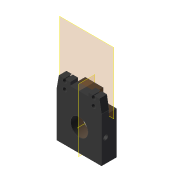
# Autodesk Inventor part: 30_Cube_Z_Focus_MGN_NEMA_adapter_M12
Saved by Autodesk Inventor 2019.4 (Build 234330000, 330)
## iProperties
Created: 2021-04-25
Part Number: 30_Cube_Z_Focus_MGN_NEMA_adapter_M12
Material: Generic
Document SubType Name: Modeling
Designer: diederichbenedict
Density: 1 g/cm^3
Appearance: Default
Author: diederichbenedict
Autodesk Inventor part; units mm, degrees
note: some values were not read from the file. Chosen so that the rebuilt part matches the saved one: sketch regions of "Extrusion1".
ref_plane "YZ Plane" through (0, 0, 0) normal (1, 0, 0) x (0, 1, 0)
ref_plane "XZ Plane" through (0, 0, 0) normal (0, 1, 0) x (-1, 0, 0)
ref_plane "XY Plane" through (0, 0, 0) normal (0, 0, 1) x (1, 0, 0)
ref_plane "Work Plane1" through (0, 0, 0) normal (0, 0, 1) x (1, 0, 0)
sketch "Sketch1" plane through (0, 0, 0) normal (0, 0, 1) x (1, 0, 0)
  circle A0 centre (6.843, -28.9967) radius 1.4 projected
  circle A1 centre (26.1569, -28.9967) radius 1.4 projected
  circle A2 centre (26.1569, -23.9967) radius 1.4 projected
  circle A3 centre (6.843, -23.9967) radius 1.4 projected
  line L0 (0.4643, -12) -> (0, -12) construction
  line L1 (3.1567, -14.6923) -> (0.4643, -12) construction
  line L2 (3.1567, -32.6831) -> (3.1567, -14.6923) construction
  line L3 (10.5294, -32.6831) -> (3.1567, -32.6831) projected
  line L4 (10.5294, -14.6923) -> (10.5294, -32.6831) construction
  line L5 (9, -11) -> (10.5294, -14.6923) construction
  line L6 (2.8, -11) -> (9, -11) construction
  line L7 (2.8, 0) -> (2.8, -11) construction
  line L8 (30.2, 0) -> (2.8, 0) construction
  line L9 (30.2, 0) -> (30.2, -11) construction
  line L10 (24, -11) -> (30.2, -11) construction
  line L11 (24, -11) -> (22.4706, -14.6923) construction
  line L12 (22.4706, -14.6923) -> (22.4706, -32.6831) construction
  line L13 (22.4706, -32.6831) -> (29.8433, -32.6831) projected
  line L14 (29.8433, -32.6831) -> (29.8433, -14.6923) construction
  line L15 (29.8433, -14.6923) -> (32.5357, -12) construction
  line L16 (33, -12) -> (32.5357, -12) construction
  line L17 (33, -12) -> (33, 5) construction
  line L18 (0, 5) -> (0, -12) construction
  circle A4 centre (16.4744, -46.03) radius 10 projected
  circle A5 centre (16.4744, -46.03) radius 12.5
  line L19 (31.4744, -31.03) -> (1.4744, -31.03) construction
  line L20 (1.4744, -31.03) -> (1.4744, -61.03) construction
  line L21 (1.4744, -61.03) -> (31.4744, -61.03) construction
  line L22 (31.4744, -61.03) -> (31.4744, -31.03) construction
  line L23 (31.4744, -31.03) -> (1.4744, -61.03) construction
  line L24 (1.4744, -31.03) -> (31.4744, -61.03) construction
  line L25 (31.4744, -61.03) -> (1.4744, -61.03)
  line L26 (1.4744, -61.03) -> (1.4744, -31.03)
  line L27 (1.4744, -31.03) -> (31.4744, -31.03)
  line L28 (31.4744, -31.03) -> (31.4744, -61.03)
  line L29 (31.4744, -61.03) -> (1.4744, -31.03) construction
  line L30 (1.4744, -61.03) -> (31.4744, -31.03) construction
  line L31 (1.4744, -31.03) -> (3.1567, -21.6555)
  line L32 (3.1567, -21.6555) -> (29.8433, -21.6555)
  line L33 (31.4744, -31.03) -> (29.8433, -21.6555)
  circle A6 centre (15.4444, 14.8) radius 2 projected
  line L34 (19.4444, 18.8) -> (33, 5) projected
  line L35 (11.4444, 18.8) -> (19.4444, 18.8) projected
  line L36 (0, 5) -> (11.4444, 18.8) projected
  circle A7 centre (3.9444, 3.3) radius 1.45 projected
  circle A8 centre (26.9444, 3.3) radius 1.45 projected
  point P0 (0, 0)
  dimension "d0" = 25
  dimension "d1" = 30
  dimension "d2" = 30
  constraints: 30 end point, 4 midpoint, 4 parallel, 3 perpendicular, 2 horizontal, 2 point on line, 1 centre point, 1 coincident
  measures "d0" diameter of A5
  measures "d1" distance of L21.end L20.end
  measures "d2" distance of L20.end L19.end
extrude "Extrusion1" add sketch "Sketch1" along normal blind 5 contours L25 L26 L27 L28 | L27 L31 L32 L33
sketch "Sketch2" plane through (0, 0, 0) normal (0, 0, -1) x (-1, 0, 0)
  circle A0 centre (-16.4744, -46.03) radius 12.5 projected
  circle A1 centre (-16.4744, -46.03) radius 10.5
  line L0 (0.4956, -63) -> (-33.4444, -63) projected
  circle A2 centre (-16.4744, -46.03) radius 12.5 projected
  arc A3 (-23.9744, -56.03) -> (-8.9744, -56.03) centre (-16.4744, -46.03) ccw
  arc A4 (-21.3847, -34.5348) -> (-28.8847, -47.5252) centre (-16.4744, -46.03) ccw
  arc A5 (-4.0642, -47.5252) -> (-11.5642, -34.5348) centre (-16.4744, -46.03) ccw
  point P0 (0, 0)
  dimension "d5" = 21
  constraints: 12 point on circle, 4 centre point, 2 coincident, 3 other
  measures "d5" diameter of A1
extrude "Extrusion2" add sketch "Sketch2" against normal up to surface (5 mm away)
sketch "Sketch3" plane through (0, 0, 0) normal (0, 0, -1) x (-1, 0, 0)
  line L0 (-30.5357, -14) -> (-24, -14) construction
  line L1 (-30.5357, -14) -> (-29.8433, -14.6923) construction
  line L2 (-29.8433, -14.6923) -> (-29.8433, -32.6831) construction
  line L3 (-29.8433, -32.6831) -> (-22.4706, -32.6831) projected
  line L4 (-22.4706, -32.6831) -> (-10.5294, -32.6831)
  line L5 (-10.5294, -32.6831) -> (-10.5294, -22.0651)
  line L6 (-10.5294, -22.0651) -> (-22.4706, -22.0651)
  line L7 (-22.4706, -22.0651) -> (-22.4706, -32.6831)
  circle A0 centre (-6.843, -23.9967) radius 1.4 construction
  circle A1 centre (-26.1569, -23.9967) radius 1.4 construction
  circle A2 centre (-26.1569, -28.9967) radius 1.4 construction
  circle A3 centre (-6.843, -28.9967) radius 1.4 construction
  line L8 (-3.1567, -21.6555) -> (-1.4744, -31.03) construction
  line L9 (-29.8433, -21.6555) -> (-3.1567, -21.6555) construction
  line L10 (-31.4744, -31.03) -> (-29.8433, -21.6555) construction
  line L11 (-31.4744, -61.03) -> (-31.4744, -31.03) construction
  line L12 (-1.4744, -61.03) -> (-31.4744, -61.03) projected
  line L13 (-1.4744, -31.03) -> (-1.4744, -61.03) construction
  line L14 (-31.4744, -32.6831) -> (-29.8433, -32.6831)
  line L15 (-3.1567, -32.6831) -> (-1.4744, -32.6831)
  line L16 (-31.4744, -61.03) -> (-1.4744, -61.03)
  line L17 (-1.4744, -61.03) -> (-1.4744, -32.6831)
  line L18 (-1.4744, -32.6831) -> (-31.4744, -32.6831)
  line L19 (-31.4744, -32.6831) -> (-31.4744, -61.03)
  circle A4 centre (-26.1569, -28.9967) radius 1.4 projected
  circle A5 centre (-26.1569, -23.9967) radius 1.4 projected
  line L20 (-24, -14) -> (-24, -11) projected
  line L21 (-22.4706, -32.6831) -> (-22.4706, -14.6923) projected
  line L22 (-22.4706, -14.6923) -> (-24, -11) projected
  circle A6 centre (-16.4256, -45.91) radius 10.6939 projected
  point P0 (0, 0)
  constraints: 20 end point, 4 parallel, 4 point on line, 2 horizontal, 2 perpendicular, 1 collinear
extrude "Extrusion4" add sketch "Sketch3" along normal blind 5 contours L3 L4 L18 L15 L17 L12 L19 L14 | L7 L6 L5 L4
sketch "Sketch4" plane through (3.1567, -21.6555, 0) normal (0, 1, 0) x (1, 0, 0)
  line L0 (-6.8596, 8.2929) -> (32.2101, 8.2929)
  line L1 (32.2101, 8.2929) -> (32.2101, -9.1799)
  line L2 (32.2101, -9.1799) -> (-6.8596, -9.1799)
  line L3 (-6.8596, -9.1799) -> (-6.8596, 8.2929)
  point P0 (-3.1567, 0)
  constraints: 8 end point, 2 parallel, 1 horizontal, 1 perpendicular
extrude "Extrusion5" cut sketch "Sketch4" against normal blind 1
sketch "Sketch5" plane through (0, 0, 5) normal (0, 0, 1) x (1, 0, 0)
  circle A0 centre (6.843, -28.9967) radius 1.4 projected
  circle A1 centre (26.1569, -28.9967) radius 1.4 projected
  line L0 (25.7553, -22.6555) -> (7.2447, -22.6555) projected
  arc A2 (6.4414, -22.6555) -> (7.2447, -22.6555) centre (6.843, -23.9967) ccw projected
  line L1 (6.4414, -22.6555) -> (2.9772, -22.6555) projected
  line L2 (2.9772, -22.6555) -> (1.4744, -31.03) projected
  line L3 (1.4744, -31.03) -> (1.4744, -61.03) projected
  line L4 (1.4744, -61.03) -> (31.4744, -61.03) projected
  line L5 (31.4744, -61.03) -> (31.4744, -31.03) projected
  line L6 (31.4744, -31.03) -> (30.0173, -22.6555) projected
  line L7 (30.0173, -22.6555) -> (26.5586, -22.6555) projected
  arc A3 (25.7553, -22.6555) -> (26.5586, -22.6555) centre (26.1569, -23.9967) ccw projected
  line L8 (10.5294, -20.3437) -> (22.4706, -20.3437)
  line L9 (22.4706, -20.3437) -> (22.4706, -24.9674)
  line L10 (22.4706, -24.9674) -> (10.5294, -24.9674)
  line L11 (10.5294, -24.9674) -> (10.5294, -20.3437)
  line L12 (10.5294, -22.6555) -> (22.4706, -22.6555) projected
  line L13 (10.5294, -20.3437) -> (22.4706, -24.9674) construction
  line L14 (22.4706, -20.3437) -> (10.5294, -24.9674) construction
  point P0 (0, 0)
  point P1 (16.5, -22.6555)
  constraints: 12 end point, 3 midpoint, 3 parallel, 1 perpendicular
extrude "Extrusion6" cut sketch "Sketch5" against normal through all contours L9 L10 L11 L0 | L0 L11 L8 L9
ref_plane "Work Plane2" through (16.4744, -61.03, 5) normal (1, 0, 0) x (0, 0, -1)
sketch "Sketch6" plane through (16.4744, -61.03, 5) normal (1, 0, 0) x (0, 0, -1)
  line L0 (0, 5.17) -> (0.15, 5.17)
  line L1 (0, 5.17) -> (0.15, 5.17) construction
  line L2 (0.15, 5.17) -> (0.3567, 4.812)
  line L3 (0.3567, 4.812) -> (0.5067, 4.812)
  line L4 (0.5067, 4.812) -> (0.7133, 5.17)
  line L5 (0.7133, 5.17) -> (0.7133, 4.17)
  line L6 (0.7133, 4.17) -> (0, 4.17)
  line L7 (0, 4.17) -> (0, 5.17)
  line L8 (-2, 15.12) -> (12, 15.12) projected
  point P0 (5, 61.03)
  point P1 (0, 0)
  dimension "d16" = 0.15
  dimension "d17" = 0
  dimension "d18" = 120
  dimension "d19" = 0.15
  dimension "d20" = 120
  dimension "d21" = 1
  dimension "d22" = 0.7133
  dimension "d33" = 9.95
  constraints: 16 end point, 3 perpendicular, 2 horizontal, 1 collinear, 1 parallel, 1 point on line
  measures "d16" distance of L0.start L0.end
  measures "d17" distance between parallel lines of L0 L1
  measures "d18" angle of L0 L2
  measures "d19" distance of L2.end L3.end
  measures "d20" angle of L4 L3
  measures "d21" distance of L4.end L5.end
  measures "d22" distance between parallel lines of L7 L5
  measures "d33" distance from line of L8 L4.end
coil "Coil1" sketch "Sketch6" operation add axis through (16.4744, -45.91, 0) along (0, 0, -1) pitch 0.7133 turns 13 hand right
sketch "Sketch7" plane through (0, 0, 5) normal (0, 0, 1) x (1, 0, 0)
  circle A0 centre (16.4744, -46.03) radius 10.5 projected
  circle A1 centre (16.4744, -46.03) radius 6
  point P0 (0, 0)
  point P1 (16.4744, -56.53)
  dimension "d34" = 12
  constraints: 1 centre point, 1 coincident, 1 vertical alignment
  measures "d34" diameter of A1
extrude "Extrusion7" add sketch "Sketch7" against normal blind 0.3
sketch "Sketch8" plane through (0, 0, -5) normal (0, 0, -1) x (-1, 0, 0)
  circle A0 centre (-16.4256, -45.91) radius 10.6939 projected
  circle A1 centre (-16.4256, -45.91) radius 8.8
  point P0 (0, 0)
  dimension "d37" = 17.6
  constraints: 1 centre point, 1 coincident
  measures "d37" diameter of A1
extrude "Extrusion8" add sketch "Sketch8" against normal up to surface (9.7 mm away)
sketch "Sketch9" plane through (31.4744, -61.03, 5) normal (1, 0, 0) x (0, 0, -1)
  line L0 (0.3, 6.32) -> (0.3, 23.92) projected
  line L1 (10, 23.92) -> (10, 6.32) projected
  circle A0 centre (2.8356, 15.12) radius 1.45
  point P0 (5, 61.03)
  dimension "d40" = 2.9
  constraints: 1 centre point
  measures "d40" diameter of A0
extrude "Extrusion9" cut sketch "Sketch9" against normal through all
equation "\"d19\" = d16"
equation "\"d20\" = d18"
body "Solid1"
